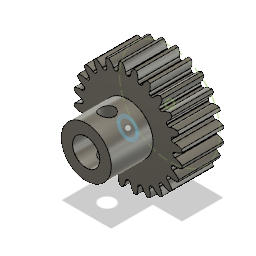
GearHægriVinstri v1 (Autodesk Fusion 360 design; units mm, degrees)
description: Spur Gear; Module: 1.000000; Num Teeth: 24; Pressure Angle: 20.000000; Backlash: 0.00 mm
Autodesk Fusion 360 part; units mm, degrees
(part 1 of 5)
sketch "Sketch1" plane through (0, 0, 0) normal (0, 0, 1) x (1, 0, 0)
  circle A0 centre (0, 0) radius 10.7492
  circle A1 centre (0, 0) radius 2
extrude "Extrude1" add sketch "Sketch1" along normal blind 2
sketch "Sketch2" plane through (0, 0, 0) normal (0, 0, 1) x (1, 0, 0)
  spline S0 degree 5 poles (11.2399, -0.9051) (11.2449, -0.9055) (11.255, -0.9062) (11.27, -0.9068) (11.2901, -0.907) (11.3152, -0.9062) (11.3404, -0.9047) (11.3655, -0.9028) (11.3907, -0.9006) (11.416, -0.8982) (11.4412, -0.8957) (11.4664, -0.8929) (11.4917, -0.8899) (11.5169, -0.8866) (11.5422, -0.8828) (11.5674, -0.8788) (11.5927, -0.8745) (11.6179, -0.87) (11.6432, -0.8652) (11.6685, -0.8603) (11.6937, -0.8552) (11.719, -0.8499) (11.7443, -0.8443) (11.7695, -0.8386) (11.7948, -0.8327) (11.82, -0.8265) (11.8453, -0.8202) (11.8706, -0.8136) (11.8958, -0.8069) (11.921, -0.8) (11.9463, -0.7929) (11.9715, -0.7857) (11.9967, -0.7783) (12.0219, -0.7707) (12.0471, -0.7629) (12.0723, -0.755) (12.0975, -0.7469) (12.1227, -0.7387) (12.1479, -0.7302) (12.173, -0.7217) (12.1982, -0.7129) (12.2233, -0.7041) (12.2484, -0.695) (12.2735, -0.6858) (12.2986, -0.6765) (12.3237, -0.667) (12.3488, -0.6573) (12.3739, -0.6475) (12.3989, -0.6376) (12.424, -0.6275) (12.449, -0.6173) (12.474, -0.6069) (12.499, -0.5964) (12.5239, -0.5858) (12.5489, -0.575) (12.5738, -0.564) (12.5988, -0.553) (12.6237, -0.5418) (12.6486, -0.5304) (12.6735, -0.5189) (12.6983, -0.5073) (12.7232, -0.4956) (12.748, -0.4837) (12.7728, -0.4717) (12.7976, -0.4595) (12.8223, -0.4473) (12.8471, -0.4349) (12.8718, -0.4223) (12.8965, -0.4097) (12.9212, -0.3969) (12.9458, -0.384) (12.9655, -0.3735) (12.9803, -0.3657) (12.9902, -0.3604) (12.9951, -0.3577) knots 0 0 0 0 0 0 0.01428571 0.02857143 0.04285714 0.05714286 0.07142857 0.08571429 0.1 0.11428571 0.12857143 0.14285714 0.15714286 0.17142857 0.18571429 0.2 0.21428571 0.22857143 0.24285714 0.25714286 0.27142857 0.28571429 0.3 0.31428571 0.32857143 0.34285714 0.35714286 0.37142857 0.38571429 0.4 0.41428571 0.42857143 0.44285714 0.45714286 0.47142857 0.48571429 0.5 0.51428571 0.52857143 0.54285714 0.55714286 0.57142857 0.58571429 0.6 0.61428571 0.62857143 0.64285714 0.65714286 0.67142857 0.68571429 0.7 0.71428571 0.72857143 0.74285714 0.75714286 0.77142857 0.78571429 0.8 0.81428571 0.82857143 0.84285714 0.85714286 0.87142857 0.88571429 0.9 0.91428571 0.92857143 0.94285714 0.95714286 0.97142857 0.98571429 1 1 1 1 1 1
  spline S1 degree 5 poles (11.2399, 0.9051) (11.2449, 0.9055) (11.255, 0.9062) (11.27, 0.9068) (11.2901, 0.907) (11.3152, 0.9062) (11.3404, 0.9047) (11.3655, 0.9028) (11.3907, 0.9006) (11.416, 0.8982) (11.4412, 0.8957) (11.4664, 0.8929) (11.4917, 0.8899) (11.5169, 0.8866) (11.5422, 0.8828) (11.5674, 0.8788) (11.5927, 0.8745) (11.6179, 0.87) (11.6432, 0.8652) (11.6685, 0.8603) (11.6937, 0.8552) (11.719, 0.8499) (11.7443, 0.8443) (11.7695, 0.8386) (11.7948, 0.8327) (11.82, 0.8265) (11.8453, 0.8202) (11.8706, 0.8136) (11.8958, 0.8069) (11.921, 0.8) (11.9463, 0.7929) (11.9715, 0.7857) (11.9967, 0.7783) (12.0219, 0.7707) (12.0471, 0.7629) (12.0723, 0.755) (12.0975, 0.7469) (12.1227, 0.7387) (12.1479, 0.7302) (12.173, 0.7217) (12.1982, 0.7129) (12.2233, 0.7041) (12.2484, 0.695) (12.2735, 0.6858) (12.2986, 0.6765) (12.3237, 0.667) (12.3488, 0.6573) (12.3739, 0.6475) (12.3989, 0.6376) (12.424, 0.6275) (12.449, 0.6173) (12.474, 0.6069) (12.499, 0.5964) (12.5239, 0.5858) (12.5489, 0.575) (12.5738, 0.564) (12.5988, 0.553) (12.6237, 0.5418) (12.6486, 0.5304) (12.6735, 0.5189) (12.6983, 0.5073) (12.7232, 0.4956) (12.748, 0.4837) (12.7728, 0.4717) (12.7976, 0.4595) (12.8223, 0.4473) (12.8471, 0.4349) (12.8718, 0.4223) (12.8965, 0.4097) (12.9212, 0.3969) (12.9458, 0.384) (12.9655, 0.3735) (12.9803, 0.3657) (12.9902, 0.3604) (12.9951, 0.3577) knots 0 0 0 0 0 0 0.01428571 0.02857143 0.04285714 0.05714286 0.07142857 0.08571429 0.1 0.11428571 0.12857143 0.14285714 0.15714286 0.17142857 0.18571429 0.2 0.21428571 0.22857143 0.24285714 0.25714286 0.27142857 0.28571429 0.3 0.31428571 0.32857143 0.34285714 0.35714286 0.37142857 0.38571429 0.4 0.41428571 0.42857143 0.44285714 0.45714286 0.47142857 0.48571429 0.5 0.51428571 0.52857143 0.54285714 0.55714286 0.57142857 0.58571429 0.6 0.61428571 0.62857143 0.64285714 0.65714286 0.67142857 0.68571429 0.7 0.71428571 0.72857143 0.74285714 0.75714286 0.77142857 0.78571429 0.8 0.81428571 0.82857143 0.84285714 0.85714286 0.87142857 0.88571429 0.9 0.91428571 0.92857143 0.94285714 0.95714286 0.97142857 0.98571429 1 1 1 1 1 1
  arc A0 (12.9951, -0.3577) -> (12.9951, 0.3577) centre (0, 0) ccw
  line L0 (10.7045, -0.8628) -> (11.2399, -0.9051)
  line L1 (10.7045, 0.8628) -> (11.2399, 0.9051)
  line L2 (10.7045, -0.8628) -> (10.7045, 0.8628)
  point P0 (11.3636, -0.9028)
  point P1 (11.4881, -0.8903)
  point P2 (11.6131, -0.8708)
  point P3 (11.7384, -0.8456)
  point P4 (11.8639, -0.8153)
  point P5 (11.9897, -0.7803)
  point P6 (12.1155, -0.741)
  point P7 (12.2414, -0.6975)
  point P8 (12.3673, -0.6501)
  point P9 (12.4932, -0.5988)
  point P10 (12.6189, -0.5439)
  point P11 (12.7445, -0.4853)
  point P12 (12.8699, -0.4232)
  point P13 (11.3636, 0.9028)
  point P14 (11.4881, 0.8903)
  point P15 (11.6131, 0.8708)
  point P16 (11.7384, 0.8456)
  point P17 (11.8639, 0.8153)
  point P18 (11.9897, 0.7803)
  point P19 (12.1155, 0.741)
  point P20 (12.2414, 0.6975)
  point P21 (12.3673, 0.6501)
  point P22 (12.4932, 0.5988)
  point P23 (12.6189, 0.5439)
  point P24 (12.7445, 0.4853)
  point P25 (12.8699, 0.4232)
extrude "Extrude2" add sketch "Sketch2" along normal blind 2
fillet "Fillet1" radius 0.5 2 edges at (10.7145, -0.8636, 1) (10.7145, 0.8636, 1)
pattern_circular "C-Pattern1" count 24 over 360 about axis through (0, 0, 0) along (0, 0, 1) of "Extrude2", "Fillet1"
sketch "Sketch3" plane through (0, 0, 0) normal (0, 0, 1) x (1, 0, 0)
  circle A0 centre (0, 0) radius 12 construction
move_body "Move1" bodies 1 to x (0.994522, -0.104528, 0) y (0.104528, 0.994522, 0) z (0, 0, 1) at (0, 0, 0)
move_body "Move2" bodies 1 to x (0.999848, -0.017452, 0) y (0.017452, 0.999848, 0) z (0, 0, 1) at (0, 0, 0)
move_body "Move3" bodies 1 to x (0.999998, -0.001745, 0) y (0.001745, 0.999998, 0) z (0, 0, 1) at (0, 0, 0)
move_body "Move4" bodies 1 to x (0.999962, -0.008727, 0) y (0.008727, 0.999962, 0) z (0, 0, 1) at (0, 0, 0)
move_body "Move5" bodies 1 to x (0.999994, 0.003491, 0) y (-0.003491, 0.999994, 0) z (0, 0, 1) at (0, 0, 0)
move_body "Move6" bodies 1 to x (0.999998, -0.001745, 0) y (0.001745, 0.999998, 0) z (0, 0, 1) at (0, 0, 0)
extrude "Extrude3" add 1 faces at (4.7398, 6.177, 2) along direction (0, 0, 1) blind 8
sketch "sketch 2008" plane through (-156.112, -54.0793, 10) normal (0, 0, 1) x (-1, 0, 0)
  circle A0 centre (-156.112, -54.0793) radius 2
  circle A1 centre (-156.112, -54.0793) radius 2.45
extrude "Extrude4" cut sketch "sketch 2008" against normal blind 50
sketch "sketch 2024" plane through (-92.8019, -19.9804, 10) normal (0, 0, 1) x (-1, 0, 0)
  circle A0 centre (-92.8019, -19.9804) radius 2.45
  circle A1 centre (-92.8019, -19.9804) radius 2.475
extrude "Extrude5" cut sketch "sketch 2024" against normal blind 20
sketch "Sketch4" plane through (0, 0, 10) normal (0, 0, 1) x (1, 0, 0)
  circle A0 centre (0, 0) radius 2.475
  arc A1 (10.3658, -2.8452) -> (10.3996, -2.7189) centre (0, 0) ccw
  arc A2 (10.9875, -2.3564) -> (10.3996, -2.7189) centre (10.8834, -2.8454) ccw
  line L0 (10.9875, -2.3564) -> (11.0256, -2.3645)
  spline S0 degree 5 poles (11.0256, -2.3645) (11.0305, -2.3655) (11.0404, -2.3675) (11.0552, -2.3701) (11.0751, -2.3729) (11.1001, -2.3754) (11.1253, -2.3772) (11.1505, -2.3785) (11.1757, -2.3797) (11.201, -2.3806) (11.2264, -2.3814) (11.2518, -2.382) (11.2772, -2.3823) (11.3027, -2.3822) (11.3282, -2.3818) (11.3537, -2.3811) (11.3793, -2.3802) (11.405, -2.379) (11.4307, -2.3776) (11.4564, -2.376) (11.4821, -2.3742) (11.5078, -2.3722) (11.5336, -2.3701) (11.5594, -2.3677) (11.5852, -2.3651) (11.611, -2.3623) (11.6369, -2.3593) (11.6628, -2.3561) (11.6887, -2.3527) (11.7146, -2.3492) (11.7406, -2.3455) (11.7665, -2.3416) (11.7925, -2.3375) (11.8185, -2.3333) (11.8445, -2.3289) (11.8705, -2.3243) (11.8965, -2.3196) (11.9226, -2.3147) (11.9486, -2.3096) (11.9747, -2.3044) (12.0007, -2.299) (12.0268, -2.2935) (12.0529, -2.2878) (12.079, -2.282) (12.1051, -2.276) (12.1312, -2.2698) (12.1574, -2.2636) (12.1835, -2.2571) (12.2096, -2.2505) (12.2358, -2.2438) (12.2619, -2.2369) (12.288, -2.2299) (12.3142, -2.2227) (12.3403, -2.2154) (12.3665, -2.208) (12.3927, -2.2004) (12.4188, -2.1927) (12.445, -2.1848) (12.4711, -2.1768) (12.4973, -2.1687) (12.5235, -2.1604) (12.5496, -2.152) (12.5758, -2.1435) (12.6019, -2.1348) (12.6281, -2.126) (12.6542, -2.1171) (12.6804, -2.108) (12.7065, -2.0988) (12.7327, -2.0895) (12.7588, -2.08) (12.785, -2.0705) (12.8059, -2.0627) (12.8215, -2.0568) (12.832, -2.0528) (12.8372, -2.0509) knots 0 0 0 0 0 0 0.01428571 0.02857143 0.04285714 0.05714286 0.07142857 0.08571429 0.1 0.11428571 0.12857143 0.14285714 0.15714286 0.17142857 0.18571429 0.2 0.21428571 0.22857143 0.24285714 0.25714286 0.27142857 0.28571429 0.3 0.31428571 0.32857143 0.34285714 0.35714286 0.37142857 0.38571429 0.4 0.41428571 0.42857143 0.44285714 0.45714286 0.47142857 0.48571429 0.5 0.51428571 0.52857143 0.54285714 0.55714286 0.57142857 0.58571429 0.6 0.61428571 0.62857143 0.64285714 0.65714286 0.67142857 0.68571429 0.7 0.71428571 0.72857143 0.74285714 0.75714286 0.77142857 0.78571429 0.8 0.81428571 0.82857143 0.84285714 0.85714286 0.87142857 0.88571429 0.9 0.91428571 0.92857143 0.94285714 0.95714286 0.97142857 0.98571429 1 1 1 1 1 1
  arc A3 (12.8372, -2.0509) -> (12.9306, -1.3415) centre (0, 0) ccw
  spline S1 degree 5 poles (12.9306, -1.3415) (12.9261, -1.3383) (12.917, -1.3317) (12.9034, -1.322) (12.8852, -1.3091) (12.8624, -1.2931) (12.8396, -1.2772) (12.8168, -1.2614) (12.7939, -1.2457) (12.771, -1.2302) (12.7481, -1.2148) (12.7251, -1.1995) (12.702, -1.1844) (12.679, -1.1694) (12.6559, -1.1545) (12.6328, -1.1397) (12.6096, -1.1251) (12.5864, -1.1106) (12.5632, -1.0962) (12.5399, -1.082) (12.5166, -1.0679) (12.4933, -1.054) (12.4699, -1.0401) (12.4465, -1.0265) (12.423, -1.0129) (12.3996, -0.9995) (12.3761, -0.9862) (12.3525, -0.9731) (12.329, -0.9601) (12.3054, -0.9473) (12.2817, -0.9346) (12.2581, -0.9221) (12.2344, -0.9097) (12.2106, -0.8974) (12.1869, -0.8853) (12.1631, -0.8734) (12.1392, -0.8616) (12.1154, -0.85) (12.0915, -0.8385) (12.0676, -0.8272) (12.0436, -0.8161) (12.0197, -0.8051) (11.9957, -0.7943) (11.9716, -0.7836) (11.9476, -0.7731) (11.9235, -0.7628) (11.8993, -0.7527) (11.8752, -0.7428) (11.851, -0.733) (11.8268, -0.7234) (11.8026, -0.714) (11.7783, -0.7048) (11.754, -0.6958) (11.7297, -0.687) (11.7053, -0.6785) (11.6809, -0.6701) (11.6565, -0.6619) (11.6321, -0.6539) (11.6076, -0.6461) (11.5832, -0.6386) (11.5586, -0.6313) (11.5341, -0.6243) (11.5095, -0.6177) (11.4849, -0.6114) (11.4602, -0.6053) (11.4355, -0.5996) (11.4108, -0.5939) (11.3861, -0.5885) (11.3614, -0.5833) (11.3367, -0.5785) (11.3119, -0.5744) (11.2919, -0.572) (11.2769, -0.5706) (11.2669, -0.57) (11.2619, -0.5697) knots -1 -1 -1 -1 -1 -1 -0.98571429 -0.97142857 -0.95714286 -0.94285714 -0.92857143 -0.91428571 -0.9 -0.88571429 -0.87142857 -0.85714286 -0.84285714 -0.82857143 -0.81428571 -0.8 -0.78571429 -0.77142857 -0.75714286 -0.74285714 -0.72857143 -0.71428571 -0.7 -0.68571429 -0.67142857 -0.65714286 -0.64285714 -0.62857143 -0.61428571 -0.6 -0.58571429 -0.57142857 -0.55714286 -0.54285714 -0.52857143 -0.51428571 -0.5 -0.48571429 -0.47142857 -0.45714286 -0.44285714 -0.42857143 -0.41428571 -0.4 -0.38571429 -0.37142857 -0.35714286 -0.34285714 -0.32857143 -0.31428571 -0.3 -0.28571429 -0.27142857 -0.25714286 -0.24285714 -0.22857143 -0.21428571 -0.2 -0.18571429 -0.17142857 -0.15714286 -0.14285714 -0.12857143 -0.11428571 -0.1 -0.08571429 -0.07142857 -0.05714286 -0.04285714 -0.02857143 -0.01428571 0 0 0 0 0 0
  line L1 (11.2619, -0.5697) -> (11.223, -0.5677)
  arc A4 (10.749, -0.0653) -> (11.223, -0.5677) centre (11.249, -0.0684) ccw
  arc A5 (10.749, -0.0653) -> (10.749, 0.0653) centre (0, 0) ccw
  arc A6 (11.223, 0.5677) -> (10.749, 0.0653) centre (11.249, 0.0684) ccw
  line L2 (11.223, 0.5677) -> (11.2619, 0.5697)
  spline S2 degree 5 poles (11.2619, 0.5697) (11.2669, 0.57) (11.2769, 0.5706) (11.2919, 0.572) (11.3119, 0.5744) (11.3367, 0.5785) (11.3614, 0.5833) (11.3861, 0.5885) (11.4108, 0.5939) (11.4355, 0.5996) (11.4602, 0.6053) (11.4849, 0.6114) (11.5095, 0.6177) (11.5341, 0.6243) (11.5586, 0.6313) (11.5832, 0.6386) (11.6076, 0.6461) (11.6321, 0.6539) (11.6565, 0.6619) (11.6809, 0.6701) (11.7053, 0.6785) (11.7297, 0.687) (11.754, 0.6958) (11.7783, 0.7048) (11.8026, 0.714) (11.8268, 0.7234) (11.851, 0.733) (11.8752, 0.7428) (11.8993, 0.7527) (11.9235, 0.7628) (11.9476, 0.7731) (11.9716, 0.7836) (11.9957, 0.7943) (12.0197, 0.8051) (12.0436, 0.8161) (12.0676, 0.8272) (12.0915, 0.8385) (12.1154, 0.85) (12.1392, 0.8616) (12.1631, 0.8734) (12.1869, 0.8853) (12.2106, 0.8974) (12.2344, 0.9097) (12.2581, 0.9221) (12.2817, 0.9346) (12.3054, 0.9473) (12.329, 0.9601) (12.3525, 0.9731) (12.3761, 0.9862) (12.3996, 0.9995) (12.423, 1.0129) (12.4465, 1.0265) (12.4699, 1.0401) (12.4933, 1.054) (12.5166, 1.0679) (12.5399, 1.082) (12.5632, 1.0962) (12.5864, 1.1106) (12.6096, 1.1251) (12.6328, 1.1397) (12.6559, 1.1545) (12.679, 1.1694) (12.702, 1.1844) (12.7251, 1.1995) (12.7481, 1.2148) (12.771, 1.2302) (12.7939, 1.2457) (12.8168, 1.2614) (12.8396, 1.2772) (12.8624, 1.2931) (12.8852, 1.3091) (12.9034, 1.322) (12.917, 1.3317) (12.9261, 1.3383) (12.9306, 1.3415) knots 0 0 0 0 0 0 0.01428571 0.02857143 0.04285714 0.05714286 0.07142857 0.08571429 0.1 0.11428571 0.12857143 0.14285714 0.15714286 0.17142857 0.18571429 0.2 0.21428571 0.22857143 0.24285714 0.25714286 0.27142857 0.28571429 0.3 0.31428571 0.32857143 0.34285714 0.35714286 0.37142857 0.38571429 0.4 0.41428571 0.42857143 0.44285714 0.45714286 0.47142857 0.48571429 0.5 0.51428571 0.52857143 0.54285714 0.55714286 0.57142857 0.58571429 0.6 0.61428571 0.62857143 0.64285714 0.65714286 0.67142857 0.68571429 0.7 0.71428571 0.72857143 0.74285714 0.75714286 0.77142857 0.78571429 0.8 0.81428571 0.82857143 0.84285714 0.85714286 0.87142857 0.88571429 0.9 0.91428571 0.92857143 0.94285714 0.95714286 0.97142857 0.98571429 1 1 1 1 1 1
  arc A7 (12.9306, 1.3415) -> (12.8372, 2.0509) centre (0, 0) ccw
  spline S3 degree 5 poles (12.8372, 2.0509) (12.832, 2.0528) (12.8215, 2.0568) (12.8059, 2.0627) (12.785, 2.0705) (12.7588, 2.08) (12.7327, 2.0895) (12.7065, 2.0988) (12.6804, 2.108) (12.6542, 2.1171) (12.6281, 2.126) (12.6019, 2.1348) (12.5758, 2.1435) (12.5496, 2.152) (12.5235, 2.1604) (12.4973, 2.1687) (12.4711, 2.1768) (12.445, 2.1848) (12.4188, 2.1927) (12.3927, 2.2004) (12.3665, 2.208) (12.3403, 2.2154) (12.3142, 2.2227) (12.288, 2.2299) (12.2619, 2.2369) (12.2358, 2.2438) (12.2096, 2.2505) (12.1835, 2.2571) (12.1574, 2.2636) (12.1312, 2.2698) (12.1051, 2.276) (12.079, 2.282) (12.0529, 2.2878) (12.0268, 2.2935) (12.0007, 2.299) (11.9747, 2.3044) (11.9486, 2.3096) (11.9226, 2.3147) (11.8965, 2.3196) (11.8705, 2.3243) (11.8445, 2.3289) (11.8185, 2.3333) (11.7925, 2.3375) (11.7665, 2.3416) (11.7406, 2.3455) (11.7146, 2.3492) (11.6887, 2.3527) (11.6628, 2.3561) (11.6369, 2.3593) (11.611, 2.3623) (11.5852, 2.3651) (11.5594, 2.3677) (11.5336, 2.3701) (11.5078, 2.3722) (11.4821, 2.3742) (11.4564, 2.376) (11.4307, 2.3776) (11.405, 2.379) (11.3793, 2.3802) (11.3537, 2.3811) (11.3282, 2.3818) (11.3027, 2.3822) (11.2772, 2.3823) (11.2518, 2.382) (11.2264, 2.3814) (11.201, 2.3806) (11.1757, 2.3797) (11.1505, 2.3785) (11.1253, 2.3772) (11.1001, 2.3754) (11.0751, 2.3729) (11.0552, 2.3701) (11.0404, 2.3675) (11.0305, 2.3655) (11.0256, 2.3645) knots -1 -1 -1 -1 -1 -1 -0.98571429 -0.97142857 -0.95714286 -0.94285714 -0.92857143 -0.91428571 -0.9 -0.88571429 -0.87142857 -0.85714286 -0.84285714 -0.82857143 -0.81428571 -0.8 -0.78571429 -0.77142857 -0.75714286 -0.74285714 -0.72857143 -0.71428571 -0.7 -0.68571429 -0.67142857 -0.65714286 -0.64285714 -0.62857143 -0.61428571 -0.6 -0.58571429 -0.57142857 -0.55714286 -0.54285714 -0.52857143 -0.51428571 -0.5 -0.48571429 -0.47142857 -0.45714286 -0.44285714 -0.42857143 -0.41428571 -0.4 -0.38571429 -0.37142857 -0.35714286 -0.34285714 -0.32857143 -0.31428571 -0.3 -0.28571429 -0.27142857 -0.25714286 -0.24285714 -0.22857143 -0.21428571 -0.2 -0.18571429 -0.17142857 -0.15714286 -0.14285714 -0.12857143 -0.11428571 -0.1 -0.08571429 -0.07142857 -0.05714286 -0.04285714 -0.02857143 -0.01428571 0 0 0 0 0 0
  line L3 (11.0256, 2.3645) -> (10.9875, 2.3564)
  arc A8 (10.3996, 2.7189) -> (10.9875, 2.3564) centre (10.8834, 2.8454) ccw
  arc A9 (10.3996, 2.7189) -> (10.3658, 2.8452) centre (0, 0) ccw
  arc A10 (10.6936, 3.4531) -> (10.3658, 2.8452) centre (10.848, 2.9775) ccw
  line L4 (10.6936, 3.4531) -> (10.7307, 3.4651)
  spline S4 degree 5 poles (10.7307, 3.4651) (10.7355, 3.4667) (10.745, 3.4699) (10.7591, 3.475) (10.7777, 3.4826) (10.8007, 3.4929) (10.8233, 3.5039) (10.8459, 3.5154) (10.8683, 3.527) (10.8907, 3.5389) (10.913, 3.5508) (10.9353, 3.563) (10.9575, 3.5755) (10.9795, 3.5883) (11.0014, 3.6013) (11.0232, 3.6147) (11.0449, 3.6284) (11.0665, 3.6422) (11.088, 3.6563) (11.1095, 3.6705) (11.1309, 3.6849) (11.1522, 3.6995) (11.1734, 3.7143) (11.1946, 3.7292) (11.2156, 3.7444) (11.2366, 3.7597) (11.2575, 3.7753) (11.2783, 3.791) (11.2991, 3.8068) (11.3197, 3.8229) (11.3404, 3.8391) (11.3609, 3.8554) (11.3814, 3.8719) (11.4017, 3.8886) (11.4221, 3.9054) (11.4423, 3.9223) (11.4625, 3.9395) (11.4826, 3.9567) (11.5026, 3.9741) (11.5226, 3.9917) (11.5425, 4.0094) (11.5623, 4.0272) (11.582, 4.0452) (11.6017, 4.0633) (11.6213, 4.0815) (11.6409, 4.0999) (11.6604, 4.1184) (11.6798, 4.137) (11.6991, 4.1558) (11.7184, 4.1747) (11.7376, 4.1937) (11.7567, 4.2129) (11.7758, 4.2321) (11.7948, 4.2515) (11.8137, 4.2711) (11.8326, 4.2907) (11.8514, 4.3105) (11.8701, 4.3304) (11.8887, 4.3504) (11.9073, 4.3705) (11.9259, 4.3907) (11.9443, 4.4111) (11.9627, 4.4316) (11.981, 4.4522) (11.9993, 4.4729) (12.0174, 4.4937) (12.0356, 4.5146) (12.0536, 4.5356) (12.0716, 4.5568) (12.0895, 4.578) (12.1073, 4.5994) (12.1215, 4.6166) (12.1322, 4.6295) (12.1392, 4.6382) (12.1428, 4.6425) knots 0 0 0 0 0 0 0.01428571 0.02857143 0.04285714 0.05714286 0.07142857 0.08571429 0.1 0.11428571 0.12857143 0.14285714 0.15714286 0.17142857 0.18571429 0.2 0.21428571 0.22857143 0.24285714 0.25714286 0.27142857 0.28571429 0.3 0.31428571 0.32857143 0.34285714 0.35714286 0.37142857 0.38571429 0.4 0.41428571 0.42857143 0.44285714 0.45714286 0.47142857 0.48571429 0.5 0.51428571 0.52857143 0.54285714 0.55714286 0.57142857 0.58571429 0.6 0.61428571 0.62857143 0.64285714 0.65714286 0.67142857 0.68571429 0.7 0.71428571 0.72857143 0.74285714 0.75714286 0.77142857 0.78571429 0.8 0.81428571 0.82857143 0.84285714 0.85714286 0.87142857 0.88571429 0.9 0.91428571 0.92857143 0.94285714 0.95714286 0.97142857 0.98571429 1 1 1 1 1 1
  arc A11 (12.1428, 4.6425) -> (11.869, 5.3035) centre (0, 0) ccw
  spline S5 degree 5 poles (11.869, 5.3035) (11.8634, 5.3041) (11.8523, 5.3052) (11.8356, 5.3068) (11.8134, 5.3089) (11.7857, 5.3114) (11.758, 5.3138) (11.7304, 5.316) (11.7027, 5.3181) (11.6751, 5.3201) (11.6475, 5.322) (11.62, 5.3237) (11.5925, 5.3253) (11.565, 5.3268) (11.5376, 5.3281) (11.5102, 5.3293) (11.4828, 5.3304) (11.4554, 5.3314) (11.4281, 5.3322) (11.4009, 5.3329) (11.3736, 5.3335) (11.3465, 5.3339) (11.3193, 5.3342) (11.2922, 5.3343) (11.2651, 5.3343) (11.2381, 5.3342) (11.2111, 5.3339) (11.1842, 5.3335) (11.1573, 5.333) (11.1304, 5.3323) (11.1036, 5.3315) (11.0768, 5.3305) (11.0501, 5.3294) (11.0234, 5.3281) (10.9968, 5.3267) (10.9702, 5.3252) (10.9437, 5.3234) (10.9172, 5.3216) (10.8908, 5.3196) (10.8644, 5.3174) (10.8381, 5.3151) (10.8119, 5.3126) (10.7857, 5.31) (10.7595, 5.3072) (10.7335, 5.3042) (10.7075, 5.3011) (10.6815, 5.2978) (10.6556, 5.2943) (10.6298, 5.2907) (10.604, 5.2869) (10.5783, 5.283) (10.5527, 5.2788) (10.5272, 5.2744) (10.5017, 5.2698) (10.4763, 5.2651) (10.451, 5.2601) (10.4258, 5.255) (10.4007, 5.2497) (10.3756, 5.2443) (10.3506, 5.2386) (10.3257, 5.2326) (10.301, 5.2264) (10.2763, 5.2198) (10.2519, 5.213) (10.2275, 5.2059) (10.2032, 5.1985) (10.179, 5.1911) (10.1549, 5.1834) (10.1309, 5.1756) (10.1071, 5.1673) (10.0836, 5.1585) (10.0651, 5.1506) (10.0514, 5.1443) (10.0424, 5.1398) (10.038, 5.1376) knots -1 -1 -1 -1 -1 -1 -0.98571429 -0.97142857 -0.95714286 -0.94285714 -0.92857143 -0.91428571 -0.9 -0.88571429 -0.87142857 -0.85714286 -0.84285714 -0.82857143 -0.81428571 -0.8 -0.78571429 -0.77142857 -0.75714286 -0.74285714 -0.72857143 -0.71428571 -0.7 -0.68571429 -0.67142857 -0.65714286 -0.64285714 -0.62857143 -0.61428571 -0.6 -0.58571429 -0.57142857 -0.55714286 -0.54285714 -0.52857143 -0.51428571 -0.5 -0.48571429 -0.47142857 -0.45714286 -0.44285714 -0.42857143 -0.41428571 -0.4 -0.38571429 -0.37142857 -0.35714286 -0.34285714 -0.32857143 -0.31428571 -0.3 -0.28571429 -0.27142857 -0.25714286 -0.24285714 -0.22857143 -0.21428571 -0.2 -0.18571429 -0.17142857 -0.15714286 -0.14285714 -0.12857143 -0.11428571 -0.1 -0.08571429 -0.07142857 -0.05714286 -0.04285714 -0.02857143 -0.01428571 0 0 0 0 0 0
  line L5 (10.038, 5.1376) -> (10.0032, 5.1199)
  arc A12 (9.3416, 5.3179) -> (10.0032, 5.1199) centre (9.7761, 5.5653) ccw
  arc A13 (9.3416, 5.3179) -> (9.2762, 5.4311) centre (0, 0) ccw
  arc A14 (9.4355, 6.1031) -> (9.2762, 5.4311) centre (9.7077, 5.6837) ccw
  line L6 (9.4355, 6.1031) -> (9.4682, 6.1244)
  spline S6 degree 5 poles (9.4682, 6.1244) (9.4725, 6.1271) (9.4808, 6.1327) (9.4931, 6.1413) (9.5091, 6.1534) (9.5286, 6.1693) (9.5477, 6.1858) (9.5665, 6.2027) (9.5851, 6.2198) (9.6037, 6.237) (9.6222, 6.2543) (9.6405, 6.2719) (9.6587, 6.2897) (9.6767, 6.3077) (9.6944, 6.326) (9.712, 6.3446) (9.7295, 6.3634) (9.7467, 6.3824) (9.7639, 6.4015) (9.7809, 6.4208) (9.7979, 6.4402) (9.8147, 6.4598) (9.8314, 6.4796) (9.8479, 6.4995) (9.8643, 6.5196) (9.8806, 6.5399) (9.8968, 6.5603) (9.9128, 6.5809) (9.9288, 6.6015) (9.9446, 6.6224) (9.9603, 6.6433) (9.9759, 6.6644) (9.9914, 6.6857) (10.0068, 6.707) (10.0221, 6.7285) (10.0372, 6.7502) (10.0523, 6.7719) (10.0672, 6.7938) (10.0821, 6.8158) (10.0968, 6.8379) (10.1115, 6.8602) (10.126, 6.8825) (10.1404, 6.905) (10.1548, 6.9276) (10.169, 6.9503) (10.1831, 6.9731) (10.1971, 6.996) (10.211, 7.019) (10.2249, 7.0421) (10.2386, 7.0654) (10.2522, 7.0887) (10.2657, 7.1122) (10.2792, 7.1357) (10.2925, 7.1594) (10.3057, 7.1831) (10.3189, 7.207) (10.3319, 7.231) (10.3448, 7.255) (10.3577, 7.2792) (10.3704, 7.3034) (10.3831, 7.3278) (10.3956, 7.3522) (10.4081, 7.3767) (10.4205, 7.4014) (10.4327, 7.4261) (10.4449, 7.4509) (10.457, 7.4758) (10.469, 7.5008) (10.4809, 7.5259) (10.4927, 7.551) (10.5044, 7.5763) (10.5136, 7.5966) (10.5206, 7.6118) (10.5252, 7.622) (10.5275, 7.6271) knots 0 0 0 0 0 0 0.01428571 0.02857143 0.04285714 0.05714286 0.07142857 0.08571429 0.1 0.11428571 0.12857143 0.14285714 0.15714286 0.17142857 0.18571429 0.2 0.21428571 0.22857143 0.24285714 0.25714286 0.27142857 0.28571429 0.3 0.31428571 0.32857143 0.34285714 0.35714286 0.37142857 0.38571429 0.4 0.41428571 0.42857143 0.44285714 0.45714286 0.47142857 0.48571429 0.5 0.51428571 0.52857143 0.54285714 0.55714286 0.57142857 0.58571429 0.6 0.61428571 0.62857143 0.64285714 0.65714286 0.67142857 0.68571429 0.7 0.71428571 0.72857143 0.74285714 0.75714286 0.77142857 0.78571429 0.8 0.81428571 0.82857143 0.84285714 0.85714286 0.87142857 0.88571429 0.9 0.91428571 0.92857143 0.94285714 0.95714286 0.97142857 0.98571429 1 1 1 1 1 1
  arc A15 (10.5275, 7.6271) -> (10.0919, 8.1947) centre (0, 0) ccw
  spline S7 degree 5 poles (10.0919, 8.1947) (10.0864, 8.1938) (10.0754, 8.192) (10.0589, 8.1893) (10.0369, 8.1855) (10.0094, 8.1808) (9.9821, 8.1759) (9.9548, 8.1709) (9.9275, 8.1658) (9.9004, 8.1606) (9.8732, 8.1552) (9.8462, 8.1498) (9.8192, 8.1442) (9.7923, 8.1385) (9.7654, 8.1327) (9.7386, 8.1268) (9.7119, 8.1208) (9.6852, 8.1146) (9.6587, 8.1083) (9.6321, 8.1019) (9.6057, 8.0954) (9.5793, 8.0888) (9.553, 8.0821) (9.5268, 8.0752) (9.5007, 8.0682) (9.4746, 8.0611) (9.4486, 8.0538) (9.4227, 8.0465) (9.3968, 8.039) (9.371, 8.0314) (9.3454, 8.0236) (9.3197, 8.0158) (9.2942, 8.0078) (9.2688, 7.9996) (9.2434, 7.9914) (9.2182, 7.983) (9.193, 7.9745) (9.1679, 7.9658) (9.1429, 7.9571) (9.118, 7.9482) (9.0932, 7.9391) (9.0685, 7.9299) (9.0438, 7.9206) (9.0193, 7.9111) (8.9949, 7.9015) (8.9706, 7.8918) (8.9464, 7.8819) (8.9222, 7.8718) (8.8982, 7.8616) (8.8743, 7.8513) (8.8505, 7.8408) (8.8269, 7.8302) (8.8033, 7.8193) (8.7799, 7.8083) (8.7567, 7.7972) (8.7335, 7.7858) (8.7105, 7.7744) (8.6875, 7.7627) (8.6647, 7.751) (8.6421, 7.739) (8.6196, 7.7268) (8.5973, 7.7144) (8.5752, 7.7017) (8.5533, 7.6887) (8.5316, 7.6755) (8.5101, 7.6622) (8.4887, 7.6487) (8.4673, 7.6351) (8.4462, 7.6213) (8.4253, 7.6072) (8.4049, 7.5925) (8.389, 7.5802) (8.3775, 7.5705) (8.37, 7.5639) (8.3662, 7.5605) knots -1 -1 -1 -1 -1 -1 -0.98571429 -0.97142857 -0.95714286 -0.94285714 -0.92857143 -0.91428571 -0.9 -0.88571429 -0.87142857 -0.85714286 -0.84285714 -0.82857143 -0.81428571 -0.8 -0.78571429 -0.77142857 -0.75714286 -0.74285714 -0.72857143 -0.71428571 -0.7 -0.68571429 -0.67142857 -0.65714286 -0.64285714 -0.62857143 -0.61428571 -0.6 -0.58571429 -0.57142857 -0.55714286 -0.54285714 -0.52857143 -0.51428571 -0.5 -0.48571429 -0.47142857 -0.45714286 -0.44285714 -0.42857143 -0.41428571 -0.4 -0.38571429 -0.37142857 -0.35714286 -0.34285714 -0.32857143 -0.31428571 -0.3 -0.28571429 -0.27142857 -0.25714286 -0.24285714 -0.22857143 -0.21428571 -0.2 -0.18571429 -0.17142857 -0.15714286 -0.14285714 -0.12857143 -0.11428571 -0.1 -0.08571429 -0.07142857 -0.05714286 -0.04285714 -0.02857143 -0.01428571 0 0 0 0 0 0
  line L7 (8.3662, 7.5605) -> (8.3373, 7.5344)
  arc A16 (7.6469, 7.5545) -> (8.3373, 7.5344) centre (8.0026, 7.9059) ccw
  arc A17 (7.6469, 7.5545) -> (7.5545, 7.6469) centre (0, 0) ccw
  arc A18 (7.5344, 8.3373) -> (7.5545, 7.6469) centre (7.9059, 8.0026) ccw
  line L8 (7.5344, 8.3373) -> (7.5605, 8.3662)
  spline S8 degree 5 poles (7.5605, 8.3662) (7.5639, 8.37) (7.5705, 8.3775) (7.5802, 8.389) (7.5925, 8.4049) (7.6072, 8.4253) (7.6213, 8.4462) (7.6351, 8.4673) (7.6487, 8.4887) (7.6622, 8.5101) (7.6755, 8.5316) (7.6887, 8.5533) (7.7017, 8.5752) (7.7144, 8.5973) (7.7268, 8.6196) (7.739, 8.6421) (7.751, 8.6647) (7.7627, 8.6875) (7.7744, 8.7105) (7.7858, 8.7335) (7.7972, 8.7567) (7.8083, 8.7799) (7.8193, 8.8033) (7.8302, 8.8269) (7.8408, 8.8505) (7.8513, 8.8743) (7.8616, 8.8982) (7.8718, 8.9222) (7.8819, 8.9464) (7.8918, 8.9706) (7.9015, 8.9949) (7.9111, 9.0193) (7.9206, 9.0438) (7.9299, 9.0685) (7.9391, 9.0932) (7.9482, 9.118) (7.9571, 9.1429) (7.9658, 9.1679) (7.9745, 9.193) (7.983, 9.2182) (7.9914, 9.2434) (7.9996, 9.2688) (8.0078, 9.2942) (8.0158, 9.3197) (8.0236, 9.3454) (8.0314, 9.371) (8.039, 9.3968) (8.0465, 9.4227) (8.0538, 9.4486) (8.0611, 9.4746) (8.0682, 9.5007) (8.0752, 9.5268) (8.0821, 9.553) (8.0888, 9.5793) (8.0954, 9.6057) (8.1019, 9.6321) (8.1083, 9.6587) (8.1146, 9.6852) (8.1208, 9.7119) (8.1268, 9.7386) (8.1327, 9.7654) (8.1385, 9.7923) (8.1442, 9.8192) (8.1498, 9.8462) (8.1552, 9.8732) (8.1606, 9.9004) (8.1658, 9.9275) (8.1709, 9.9548) (8.1759, 9.9821) (8.1808, 10.0094) (8.1855, 10.0369) (8.1893, 10.0589) (8.192, 10.0754) (8.1938, 10.0864) (8.1947, 10.0919) knots 0 0 0 0 0 0 0.01428571 0.02857143 0.04285714 0.05714286 0.07142857 0.08571429 0.1 0.11428571 0.12857143 0.14285714 0.15714286 0.17142857 0.18571429 0.2 0.21428571 0.22857143 0.24285714 0.25714286 0.27142857 0.28571429 0.3 0.31428571 0.32857143 0.34285714 0.35714286 0.37142857 0.38571429 0.4 0.41428571 0.42857143 0.44285714 0.45714286 0.47142857 0.48571429 0.5 0.51428571 0.52857143 0.54285714 0.55714286 0.57142857 0.58571429 0.6 0.61428571 0.62857143 0.64285714 0.65714286 0.67142857 0.68571429 0.7 0.71428571 0.72857143 0.74285714 0.75714286 0.77142857 0.78571429 0.8 0.81428571 0.82857143 0.84285714 0.85714286 0.87142857 0.88571429 0.9 0.91428571 0.92857143 0.94285714 0.95714286 0.97142857 0.98571429 1 1 1 1 1 1
  arc A19 (8.1947, 10.0919) -> (7.6271, 10.5275) centre (0, 0) ccw
  spline S9 degree 5 poles (7.6271, 10.5275) (7.622, 10.5252) (7.6118, 10.5206) (7.5966, 10.5136) (7.5763, 10.5044) (7.551, 10.4927) (7.5259, 10.4809) (7.5008, 10.469) (7.4758, 10.457) (7.4509, 10.4449) (7.4261, 10.4327) (7.4014, 10.4205) (7.3767, 10.4081) (7.3522, 10.3956) (7.3278, 10.3831) (7.3034, 10.3704) (7.2792, 10.3577) (7.255, 10.3448) (7.231, 10.3319) (7.207, 10.3189) (7.1831, 10.3057) (7.1594, 10.2925) (7.1357, 10.2792) (7.1122, 10.2657) (7.0887, 10.2522) (7.0654, 10.2386) (7.0421, 10.2249) (7.019, 10.211) (6.996, 10.1971) (6.9731, 10.1831) (6.9503, 10.169) (6.9276, 10.1548) (6.905, 10.1404) (6.8825, 10.126) (6.8602, 10.1115) (6.8379, 10.0968) (6.8158, 10.0821) (6.7938, 10.0672) (6.7719, 10.0523) (6.7502, 10.0372) (6.7285, 10.0221) (6.707, 10.0068) (6.6857, 9.9914) (6.6644, 9.9759) (6.6433, 9.9603) (6.6224, 9.9446) (6.6015, 9.9288) (6.5809, 9.9128) (6.5603, 9.8968) (6.5399, 9.8806) (6.5196, 9.8643) (6.4995, 9.8479) (6.4796, 9.8314) (6.4598, 9.8147) (6.4402, 9.7979) (6.4208, 9.7809) (6.4015, 9.7639) (6.3824, 9.7467) (6.3634, 9.7295) (6.3446, 9.712) (6.326, 9.6944) (6.3077, 9.6767) (6.2897, 9.6587) (6.2719, 9.6405) (6.2543, 9.6222) (6.237, 9.6037) (6.2198, 9.5851) (6.2027, 9.5665) (6.1858, 9.5477) (6.1693, 9.5286) (6.1534, 9.5091) (6.1413, 9.4931) (6.1327, 9.4808) (6.1271, 9.4725) (6.1244, 9.4682) knots -1 -1 -1 -1 -1 -1 -0.98571429 -0.97142857 -0.95714286 -0.94285714 -0.92857143 -0.91428571 -0.9 -0.88571429 -0.87142857 -0.85714286 -0.84285714 -0.82857143 -0.81428571 -0.8 -0.78571429 -0.77142857 -0.75714286 -0.74285714 -0.72857143 -0.71428571 -0.7 -0.68571429 -0.67142857 -0.65714286 -0.64285714 -0.62857143 -0.61428571 -0.6 -0.58571429 -0.57142857 -0.55714286 -0.54285714 -0.52857143 -0.51428571 -0.5 -0.48571429 -0.47142857 -0.45714286 -0.44285714 -0.42857143 -0.41428571 -0.4 -0.38571429 -0.37142857 -0.35714286 -0.34285714 -0.32857143 -0.31428571 -0.3 -0.28571429 -0.27142857 -0.25714286 -0.24285714 -0.22857143 -0.21428571 -0.2 -0.18571429 -0.17142857 -0.15714286 -0.14285714 -0.12857143 -0.11428571 -0.1 -0.08571429 -0.07142857 -0.05714286 -0.04285714 -0.02857143 -0.01428571 0 0 0 0 0 0
  line L9 (6.1244, 9.4682) -> (6.1031, 9.4355)
  arc A20 (5.4311, 9.2762) -> (6.1031, 9.4355) centre (5.6837, 9.7077) ccw
  arc A21 (5.4311, 9.2762) -> (5.3179, 9.3416) centre (0, 0) ccw
  arc A22 (5.1199, 10.0032) -> (5.3179, 9.3416) centre (5.5653, 9.7761) ccw
  line L10 (5.1199, 10.0032) -> (5.1376, 10.038)
  spline S10 degree 5 poles (5.1376, 10.038) (5.1398, 10.0424) (5.1443, 10.0514) (5.1506, 10.0651) (5.1585, 10.0836) (5.1673, 10.1071) (5.1756, 10.1309) (5.1834, 10.1549) (5.1911, 10.179) (5.1985, 10.2032) (5.2059, 10.2275) (5.213, 10.2519) (5.2198, 10.2763) (5.2264, 10.301) (5.2326, 10.3257) (5.2386, 10.3506) (5.2443, 10.3756) (5.2497, 10.4007) (5.255, 10.4258) (5.2601, 10.451) (5.2651, 10.4763) (5.2698, 10.5017) (5.2744, 10.5272) (5.2788, 10.5527) (5.283, 10.5783) (5.2869, 10.604) (5.2907, 10.6298) (5.2943, 10.6556) (5.2978, 10.6815) (5.3011, 10.7075) (5.3042, 10.7335) (5.3072, 10.7595) (5.31, 10.7857) (5.3126, 10.8119) (5.3151, 10.8381) (5.3174, 10.8644) (5.3196, 10.8908) (5.3216, 10.9172) (5.3234, 10.9437) (5.3252, 10.9702) (5.3267, 10.9968) (5.3281, 11.0234) (5.3294, 11.0501) (5.3305, 11.0768) (5.3315, 11.1036) (5.3323, 11.1304) (5.333, 11.1573) (5.3335, 11.1842) (5.3339, 11.2111) (5.3342, 11.2381) (5.3343, 11.2651) (5.3343, 11.2922) (5.3342, 11.3193) (5.3339, 11.3465) (5.3335, 11.3736) (5.3329, 11.4009) (5.3322, 11.4281) (5.3314, 11.4554) (5.3304, 11.4828) (5.3293, 11.5102) (5.3281, 11.5376) (5.3268, 11.565) (5.3253, 11.5925) (5.3237, 11.62) (5.322, 11.6475) (5.3201, 11.6751) (5.3181, 11.7027) (5.316, 11.7304) (5.3138, 11.758) (5.3114, 11.7857) (5.3089, 11.8134) (5.3068, 11.8356) (5.3052, 11.8523) (5.3041, 11.8634) (5.3035, 11.869) knots 0 0 0 0 0 0 0.01428571 0.02857143 0.04285714 0.05714286 0.07142857 0.08571429 0.1 0.11428571 0.12857143 0.14285714 0.15714286 0.17142857 0.18571429 0.2 0.21428571 0.22857143 0.24285714 0.25714286 0.27142857 0.28571429 0.3 0.31428571 0.32857143 0.34285714 0.35714286 0.37142857 0.38571429 0.4 0.41428571 0.42857143 0.44285714 0.45714286 0.47142857 0.48571429 0.5 0.51428571 0.52857143 0.54285714 0.55714286 0.57142857 0.58571429 0.6 0.61428571 0.62857143 0.64285714 0.65714286 0.67142857 0.68571429 0.7 0.71428571 0.72857143 0.74285714 0.75714286 0.77142857 0.78571429 0.8 0.81428571 0.82857143 0.84285714 0.85714286 0.87142857 0.88571429 0.9 0.91428571 0.92857143 0.94285714 0.95714286 0.97142857 0.98571429 1 1 1 1 1 1
  arc A23 (5.3035, 11.869) -> (4.6425, 12.1428) centre (0, 0) ccw
  spline S11 degree 5 poles (4.6425, 12.1428) (4.6382, 12.1392) (4.6295, 12.1322) (4.6166, 12.1215) (4.5994, 12.1073) (4.578, 12.0895) (4.5568, 12.0716) (4.5356, 12.0536) (4.5146, 12.0356) (4.4937, 12.0174) (4.4729, 11.9993) (4.4522, 11.981) (4.4316, 11.9627) (4.4111, 11.9443) (4.3907, 11.9259) (4.3705, 11.9073) (4.3504, 11.8887) (4.3304, 11.8701) (4.3105, 11.8514) (4.2907, 11.8326) (4.2711, 11.8137) (4.2515, 11.7948) (4.2321, 11.7758) (4.2129, 11.7567) (4.1937, 11.7376) (4.1747, 11.7184) (4.1558, 11.6991) (4.137, 11.6798) (4.1184, 11.6604) (4.0999, 11.6409) (4.0815, 11.6213) (4.0633, 11.6017) (4.0452, 11.582) (4.0272, 11.5623) (4.0094, 11.5425) (3.9917, 11.5226) (3.9741, 11.5026) (3.9567, 11.4826) (3.9395, 11.4625) (3.9223, 11.4423) (3.9054, 11.4221) (3.8886, 11.4017) (3.8719, 11.3814) (3.8554, 11.3609) (3.8391, 11.3404) (3.8229, 11.3197) (3.8068, 11.2991) (3.791, 11.2783) (3.7753, 11.2575) (3.7597, 11.2366) (3.7444, 11.2156) (3.7292, 11.1946) (3.7143, 11.1734) (3.6995, 11.1522) (3.6849, 11.1309) (3.6705, 11.1095) (3.6563, 11.088) (3.6422, 11.0665) (3.6284, 11.0449) (3.6147, 11.0232) (3.6013, 11.0014) (3.5883, 10.9795) (3.5755, 10.9575) (3.563, 10.9353) (3.5508, 10.913) (3.5389, 10.8907) (3.527, 10.8683) (3.5154, 10.8459) (3.5039, 10.8233) (3.4929, 10.8007) (3.4826, 10.7777) (3.475, 10.7591) (3.4699, 10.745) (3.4667, 10.7355) (3.4651, 10.7307) knots -1 -1 -1 -1 -1 -1 -0.98571429 -0.97142857 -0.95714286 -0.94285714 -0.92857143 -0.91428571 -0.9 -0.88571429 -0.87142857 -0.85714286 -0.84285714 -0.82857143 -0.81428571 -0.8 -0.78571429 -0.77142857 -0.75714286 -0.74285714 -0.72857143 -0.71428571 -0.7 -0.68571429 -0.67142857 -0.65714286 -0.64285714 -0.62857143 -0.61428571 -0.6 -0.58571429 -0.57142857 -0.55714286 -0.54285714 -0.52857143 -0.51428571 -0.5 -0.48571429 -0.47142857 -0.45714286 -0.44285714 -0.42857143 -0.41428571 -0.4 -0.38571429 -0.37142857 -0.35714286 -0.34285714 -0.32857143 -0.31428571 -0.3 -0.28571429 -0.27142857 -0.25714286 -0.24285714 -0.22857143 -0.21428571 -0.2 -0.18571429 -0.17142857 -0.15714286 -0.14285714 -0.12857143 -0.11428571 -0.1 -0.08571429 -0.07142857 -0.05714286 -0.04285714 -0.02857143 -0.01428571 0 0 0 0 0 0
  line L11 (3.4651, 10.7307) -> (3.4531, 10.6936)
  arc A24 (2.8452, 10.3658) -> (3.4531, 10.6936) centre (2.9775, 10.848) ccw
  arc A25 (2.8452, 10.3658) -> (2.7189, 10.3996) centre (0, 0) ccw
  arc A26 (2.3564, 10.9875) -> (2.7189, 10.3996) centre (2.8454, 10.8834) ccw
  line L12 (2.3564, 10.9875) -> (2.3645, 11.0256)
  spline S12 degree 5 poles (2.3645, 11.0256) (2.3655, 11.0305) (2.3675, 11.0404) (2.3701, 11.0552) (2.3729, 11.0751) (2.3754, 11.1001) (2.3772, 11.1253) (2.3785, 11.1505) (2.3797, 11.1757) (2.3806, 11.201) (2.3814, 11.2264) (2.382, 11.2518) (2.3823, 11.2772) (2.3822, 11.3027) (2.3818, 11.3282) (2.3811, 11.3537) (2.3802, 11.3793) (2.379, 11.405) (2.3776, 11.4307) (2.376, 11.4564) (2.3742, 11.4821) (2.3722, 11.5078) (2.3701, 11.5336) (2.3677, 11.5594) (2.3651, 11.5852) (2.3623, 11.611) (2.3593, 11.6369) (2.3561, 11.6628) (2.3527, 11.6887) (2.3492, 11.7146) (2.3455, 11.7406) (2.3416, 11.7665) (2.3375, 11.7925) (2.3333, 11.8185) (2.3289, 11.8445) (2.3243, 11.8705) (2.3196, 11.8965) (2.3147, 11.9226) (2.3096, 11.9486) (2.3044, 11.9747) (2.299, 12.0007) (2.2935, 12.0268) (2.2878, 12.0529) (2.282, 12.079) (2.276, 12.1051) (2.2698, 12.1312) (2.2636, 12.1574) (2.2571, 12.1835) (2.2505, 12.2096) (2.2438, 12.2358) (2.2369, 12.2619) (2.2299, 12.288) (2.2227, 12.3142) (2.2154, 12.3403) (2.208, 12.3665) (2.2004, 12.3927) (2.1927, 12.4188) (2.1848, 12.445) (2.1768, 12.4711) (2.1687, 12.4973) (2.1604, 12.5235) (2.152, 12.5496) (2.1435, 12.5758) (2.1348, 12.6019) (2.126, 12.6281) (2.1171, 12.6542) (2.108, 12.6804) (2.0988, 12.7065) (2.0895, 12.7327) (2.08, 12.7588) (2.0705, 12.785) (2.0627, 12.8059) (2.0568, 12.8215) (2.0528, 12.832) (2.0509, 12.8372) knots 0 0 0 0 0 0 0.01428571 0.02857143 0.04285714 0.05714286 0.07142857 0.08571429 0.1 0.11428571 0.12857143 0.14285714 0.15714286 0.17142857 0.18571429 0.2 0.21428571 0.22857143 0.24285714 0.25714286 0.27142857 0.28571429 0.3 0.31428571 0.32857143 0.34285714 0.35714286 0.37142857 0.38571429 0.4 0.41428571 0.42857143 0.44285714 0.45714286 0.47142857 0.48571429 0.5 0.51428571 0.52857143 0.54285714 0.55714286 0.57142857 0.58571429 0.6 0.61428571 0.62857143 0.64285714 0.65714286 0.67142857 0.68571429 0.7 0.71428571 0.72857143 0.74285714 0.75714286 0.77142857 0.78571429 0.8 0.81428571 0.82857143 0.84285714 0.85714286 0.87142857 0.88571429 0.9 0.91428571 0.92857143 0.94285714 0.95714286 0.97142857 0.98571429 1 1 1 1 1 1
  arc A27 (2.0509, 12.8372) -> (1.3415, 12.9306) centre (0, 0) ccw
  spline S13 degree 5 poles (1.3415, 12.9306) (1.3383, 12.9261) (1.3317, 12.917) (1.322, 12.9034) (1.3091, 12.8852) (1.2931, 12.8624) (1.2772, 12.8396) (1.2614, 12.8168) (1.2457, 12.7939) (1.2302, 12.771) (1.2148, 12.7481) (1.1995, 12.7251) (1.1844, 12.702) (1.1694, 12.679) (1.1545, 12.6559) (1.1397, 12.6328) (1.1251, 12.6096) (1.1106, 12.5864) (1.0962, 12.5632) (1.082, 12.5399) (1.0679, 12.5166) (1.054, 12.4933) (1.0401, 12.4699) (1.0265, 12.4465) (1.0129, 12.423) (0.9995, 12.3996) (0.9862, 12.3761) (0.9731, 12.3525) (0.9601, 12.329) (0.9473, 12.3054) (0.9346, 12.2817) (0.9221, 12.2581) (0.9097, 12.2344) (0.8974, 12.2106) (0.8853, 12.1869) (0.8734, 12.1631) (0.8616, 12.1392) (0.85, 12.1154) (0.8385, 12.0915) (0.8272, 12.0676) (0.8161, 12.0436) (0.8051, 12.0197) (0.7943, 11.9957) (0.7836, 11.9716) (0.7731, 11.9476) (0.7628, 11.9235) (0.7527, 11.8993) (0.7428, 11.8752) (0.733, 11.851) (0.7234, 11.8268) (0.714, 11.8026) (0.7048, 11.7783) (0.6958, 11.754) (0.687, 11.7297) (0.6785, 11.7053) (0.6701, 11.6809) (0.6619, 11.6565) (0.6539, 11.6321) (0.6461, 11.6076) (0.6386, 11.5832) (0.6313, 11.5586) (0.6243, 11.5341) (0.6177, 11.5095) (0.6114, 11.4849) (0.6053, 11.4602) (0.5996, 11.4355) (0.5939, 11.4108) (0.5885, 11.3861) (0.5833, 11.3614) (0.5785, 11.3367) (0.5744, 11.3119) (0.572, 11.2919) (0.5706, 11.2769) (0.57, 11.2669) (0.5697, 11.2619) knots -1 -1 -1 -1 -1 -1 -0.98571429 -0.97142857 -0.95714286 -0.94285714 -0.92857143 -0.91428571 -0.9 -0.88571429 -0.87142857 -0.85714286 -0.84285714 -0.82857143 -0.81428571 -0.8 -0.78571429 -0.77142857 -0.75714286 -0.74285714 -0.72857143 -0.71428571 -0.7 -0.68571429 -0.67142857 -0.65714286 -0.64285714 -0.62857143 -0.61428571 -0.6 -0.58571429 -0.57142857 -0.55714286 -0.54285714 -0.52857143 -0.51428571 -0.5 -0.48571429 -0.47142857 -0.45714286 -0.44285714 -0.42857143 -0.41428571 -0.4 -0.38571429 -0.37142857 -0.35714286 -0.34285714 -0.32857143 -0.31428571 -0.3 -0.28571429 -0.27142857 -0.25714286 -0.24285714 -0.22857143 -0.21428571 -0.2 -0.18571429 -0.17142857 -0.15714286 -0.14285714 -0.12857143 -0.11428571 -0.1 -0.08571429 -0.07142857 -0.05714286 -0.04285714 -0.02857143 -0.01428571 0 0 0 0 0 0
  line L13 (0.5697, 11.2619) -> (0.5677, 11.223)
  arc A28 (0.0653, 10.749) -> (0.5677, 11.223) centre (0.0684, 11.249) ccw
  arc A29 (0.0653, 10.749) -> (-0.0653, 10.749) centre (0, 0) ccw
  arc A30 (-0.5677, 11.223) -> (-0.0653, 10.749) centre (-0.0684, 11.249) ccw
  line L14 (-0.5677, 11.223) -> (-0.5697, 11.2619)
  spline S14 degree 5 poles (-0.5697, 11.2619) (-0.57, 11.2669) (-0.5706, 11.2769) (-0.572, 11.2919) (-0.5744, 11.3119) (-0.5785, 11.3367) (-0.5833, 11.3614) (-0.5885, 11.3861) (-0.5939, 11.4108) (-0.5996, 11.4355) (-0.6053, 11.4602) (-0.6114, 11.4849) (-0.6177, 11.5095) (-0.6243, 11.5341) (-0.6313, 11.5586) (-0.6386, 11.5832) (-0.6461, 11.6076) (-0.6539, 11.6321) (-0.6619, 11.6565) (-0.6701, 11.6809) (-0.6785, 11.7053) (-0.687, 11.7297) (-0.6958, 11.754) (-0.7048, 11.7783) (-0.714, 11.8026) (-0.7234, 11.8268) (-0.733, 11.851) (-0.7428, 11.8752) (-0.7527, 11.8993) (-0.7628, 11.9235) (-0.7731, 11.9476) (-0.7836, 11.9716) (-0.7943, 11.9957) (-0.8051, 12.0197) (-0.8161, 12.0436) (-0.8272, 12.0676) (-0.8385, 12.0915) (-0.85, 12.1154) (-0.8616, 12.1392) (-0.8734, 12.1631) (-0.8853, 12.1869) (-0.8974, 12.2106) (-0.9097, 12.2344) (-0.9221, 12.2581) (-0.9346, 12.2817) (-0.9473, 12.3054) (-0.9601, 12.329) (-0.9731, 12.3525) (-0.9862, 12.3761) (-0.9995, 12.3996) (-1.0129, 12.423) (-1.0265, 12.4465) (-1.0401, 12.4699) (-1.054, 12.4933) (-1.0679, 12.5166) (-1.082, 12.5399) (-1.0962, 12.5632) (-1.1106, 12.5864) (-1.1251, 12.6096) (-1.1397, 12.6328) (-1.1545, 12.6559) (-1.1694, 12.679) (-1.1844, 12.702) (-1.1995, 12.7251) (-1.2148, 12.7481) (-1.2302, 12.771) (-1.2457, 12.7939) (-1.2614, 12.8168) (-1.2772, 12.8396) (-1.2931, 12.8624) (-1.3091, 12.8852) (-1.322, 12.9034) (-1.3317, 12.917) (-1.3383, 12.9261) (-1.3415, 12.9306) knots 0 0 0 0 0 0 0.01428571 0.02857143 0.04285714 0.05714286 0.07142857 0.08571429 0.1 0.11428571 0.12857143 0.14285714 0.15714286 0.17142857 0.18571429 0.2 0.21428571 0.22857143 0.24285714 0.25714286 0.27142857 0.28571429 0.3 0.31428571 0.32857143 0.34285714 0.35714286 0.37142857 0.38571429 0.4 0.41428571 0.42857143 0.44285714 0.45714286 0.47142857 0.48571429 0.5 0.51428571 0.52857143 0.54285714 0.55714286 0.57142857 0.58571429 0.6 0.61428571 0.62857143 0.64285714 0.65714286 0.67142857 0.68571429 0.7 0.71428571 0.72857143 0.74285714 0.75714286 0.77142857 0.78571429 0.8 0.81428571 0.82857143 0.84285714 0.85714286 0.87142857 0.88571429 0.9 0.91428571 0.92857143 0.94285714 0.95714286 0.97142857 0.98571429 1 1 1 1 1 1
  arc A31 (-1.3415, 12.9306) -> (-2.0509, 12.8372) centre (0, 0) ccw
  spline S15 degree 5 poles (-2.0509, 12.8372) (-2.0528, 12.832) (-2.0568, 12.8215) (-2.0627, 12.8059) (-2.0705, 12.785) (-2.08, 12.7588) (-2.0895, 12.7327) (-2.0988, 12.7065) (-2.108, 12.6804) (-2.1171, 12.6542) (-2.126, 12.6281) (-2.1348, 12.6019) (-2.1435, 12.5758) (-2.152, 12.5496) (-2.1604, 12.5235) (-2.1687, 12.4973) (-2.1768, 12.4711) (-2.1848, 12.445) (-2.1927, 12.4188) (-2.2004, 12.3927) (-2.208, 12.3665) (-2.2154, 12.3403) (-2.2227, 12.3142) (-2.2299, 12.288) (-2.2369, 12.2619) (-2.2438, 12.2358) (-2.2505, 12.2096) (-2.2571, 12.1835) (-2.2636, 12.1574) (-2.2698, 12.1312) (-2.276, 12.1051) (-2.282, 12.079) (-2.2878, 12.0529) (-2.2935, 12.0268) (-2.299, 12.0007) (-2.3044, 11.9747) (-2.3096, 11.9486) (-2.3147, 11.9226) (-2.3196, 11.8965) (-2.3243, 11.8705) (-2.3289, 11.8445) (-2.3333, 11.8185) (-2.3375, 11.7925) (-2.3416, 11.7665) (-2.3455, 11.7406) (-2.3492, 11.7146) (-2.3527, 11.6887) (-2.3561, 11.6628) (-2.3593, 11.6369) (-2.3623, 11.611) (-2.3651, 11.5852) (-2.3677, 11.5594) (-2.3701, 11.5336) (-2.3722, 11.5078) (-2.3742, 11.4821) (-2.376, 11.4564) (-2.3776, 11.4307) (-2.379, 11.405) (-2.3802, 11.3793) (-2.3811, 11.3537) (-2.3818, 11.3282) (-2.3822, 11.3027) (-2.3823, 11.2772) (-2.382, 11.2518) (-2.3814, 11.2264) (-2.3806, 11.201) (-2.3797, 11.1757) (-2.3785, 11.1505) (-2.3772, 11.1253) (-2.3754, 11.1001) (-2.3729, 11.0751) (-2.3701, 11.0552) (-2.3675, 11.0404) (-2.3655, 11.0305) (-2.3645, 11.0256) knots -1 -1 -1 -1 -1 -1 -0.98571429 -0.97142857 -0.95714286 -0.94285714 -0.92857143 -0.91428571 -0.9 -0.88571429 -0.87142857 -0.85714286 -0.84285714 -0.82857143 -0.81428571 -0.8 -0.78571429 -0.77142857 -0.75714286 -0.74285714 -0.72857143 -0.71428571 -0.7 -0.68571429 -0.67142857 -0.65714286 -0.64285714 -0.62857143 -0.61428571 -0.6 -0.58571429 -0.57142857 -0.55714286 -0.54285714 -0.52857143 -0.51428571 -0.5 -0.48571429 -0.47142857 -0.45714286 -0.44285714 -0.42857143 -0.41428571 -0.4 -0.38571429 -0.37142857 -0.35714286 -0.34285714 -0.32857143 -0.31428571 -0.3 -0.28571429 -0.27142857 -0.25714286 -0.24285714 -0.22857143 -0.21428571 -0.2 -0.18571429 -0.17142857 -0.15714286 -0.14285714 -0.12857143 -0.11428571 -0.1 -0.08571429 -0.07142857 -0.05714286 -0.04285714 -0.02857143 -0.01428571 0 0 0 0 0 0
  line L15 (-2.3645, 11.0256) -> (-2.3564, 10.9875)
  arc A32 (-2.7189, 10.3996) -> (-2.3564, 10.9875) centre (-2.8454, 10.8834) ccw
  arc A33 (-2.7189, 10.3996) -> (-2.8452, 10.3658) centre (0, 0) ccw
  arc A34 (-3.4531, 10.6936) -> (-2.8452, 10.3658) centre (-2.9775, 10.848) ccw
  line L16 (-3.4531, 10.6936) -> (-3.4651, 10.7307)
  spline S16 degree 5 poles (-3.4651, 10.7307) (-3.4667, 10.7355) (-3.4699, 10.745) (-3.475, 10.7591) (-3.4826, 10.7777) (-3.4929, 10.8007) (-3.5039, 10.8233) (-3.5154, 10.8459) (-3.527, 10.8683) (-3.5389, 10.8907) (-3.5508, 10.913) (-3.563, 10.9353) (-3.5755, 10.9575) (-3.5883, 10.9795) (-3.6013, 11.0014) (-3.6147, 11.0232) (-3.6284, 11.0449) (-3.6422, 11.0665) (-3.6563, 11.088) (-3.6705, 11.1095) (-3.6849, 11.1309) (-3.6995, 11.1522) (-3.7143, 11.1734) (-3.7292, 11.1946) (-3.7444, 11.2156) (-3.7597, 11.2366) (-3.7753, 11.2575) (-3.791, 11.2783) (-3.8068, 11.2991) (-3.8229, 11.3197) (-3.8391, 11.3404) (-3.8554, 11.3609) (-3.8719, 11.3814) (-3.8886, 11.4017) (-3.9054, 11.4221) (-3.9223, 11.4423) (-3.9395, 11.4625) (-3.9567, 11.4826) (-3.9741, 11.5026) (-3.9917, 11.5226) (-4.0094, 11.5425) (-4.0272, 11.5623) (-4.0452, 11.582) (-4.0633, 11.6017) (-4.0815, 11.6213) (-4.0999, 11.6409) (-4.1184, 11.6604) (-4.137, 11.6798) (-4.1558, 11.6991) (-4.1747, 11.7184) (-4.1937, 11.7376) (-4.2129, 11.7567) (-4.2321, 11.7758) (-4.2515, 11.7948) (-4.2711, 11.8137) (-4.2907, 11.8326) (-4.3105, 11.8514) (-4.3304, 11.8701) (-4.3504, 11.8887) (-4.3705, 11.9073) (-4.3907, 11.9259) (-4.4111, 11.9443) (-4.4316, 11.9627) (-4.4522, 11.981) (-4.4729, 11.9993) (-4.4937, 12.0174) (-4.5146, 12.0356) (-4.5356, 12.0536) (-4.5568, 12.0716) (-4.578, 12.0895) (-4.5994, 12.1073) (-4.6166, 12.1215) (-4.6295, 12.1322) (-4.6382, 12.1392) (-4.6425, 12.1428) knots 0 0 0 0 0 0 0.01428571 0.02857143 0.04285714 0.05714286 0.07142857 0.08571429 0.1 0.11428571 0.12857143 0.14285714 0.15714286 0.17142857 0.18571429 0.2 0.21428571 0.22857143 0.24285714 0.25714286 0.27142857 0.28571429 0.3 0.31428571 0.32857143 0.34285714 0.35714286 0.37142857 0.38571429 0.4 0.41428571 0.42857143 0.44285714 0.45714286 0.47142857 0.48571429 0.5 0.51428571 0.52857143 0.54285714 0.55714286 0.57142857 0.58571429 0.6 0.61428571 0.62857143 0.64285714 0.65714286 0.67142857 0.68571429 0.7 0.71428571 0.72857143 0.74285714 0.75714286 0.77142857 0.78571429 0.8 0.81428571 0.82857143 0.84285714 0.85714286 0.87142857 0.88571429 0.9 0.91428571 0.92857143 0.94285714 0.95714286 0.97142857 0.98571429 1 1 1 1 1 1
  arc A35 (-4.6425, 12.1428) -> (-5.3035, 11.869) centre (0, 0) ccw
  spline S17 degree 5 poles (-5.3035, 11.869) (-5.3041, 11.8634) (-5.3052, 11.8523) (-5.3068, 11.8356) (-5.3089, 11.8134) (-5.3114, 11.7857) (-5.3138, 11.758) (-5.316, 11.7304) (-5.3181, 11.7027) (-5.3201, 11.6751) (-5.322, 11.6475) (-5.3237, 11.62) (-5.3253, 11.5925) (-5.3268, 11.565) (-5.3281, 11.5376) (-5.3293, 11.5102) (-5.3304, 11.4828) (-5.3314, 11.4554) (-5.3322, 11.4281) (-5.3329, 11.4009) (-5.3335, 11.3736) (-5.3339, 11.3465) (-5.3342, 11.3193) (-5.3343, 11.2922) (-5.3343, 11.2651) (-5.3342, 11.2381) (-5.3339, 11.2111) (-5.3335, 11.1842) (-5.333, 11.1573) (-5.3323, 11.1304) (-5.3315, 11.1036) (-5.3305, 11.0768) (-5.3294, 11.0501) (-5.3281, 11.0234) (-5.3267, 10.9968) (-5.3252, 10.9702) (-5.3234, 10.9437) (-5.3216, 10.9172) (-5.3196, 10.8908) (-5.3174, 10.8644) (-5.3151, 10.8381) (-5.3126, 10.8119) (-5.31, 10.7857) (-5.3072, 10.7595) (-5.3042, 10.7335) (-5.3011, 10.7075) (-5.2978, 10.6815) (-5.2943, 10.6556) (-5.2907, 10.6298) (-5.2869, 10.604) (-5.283, 10.5783) (-5.2788, 10.5527) (-5.2744, 10.5272) (-5.2698, 10.5017) (-5.2651, 10.4763) (-5.2601, 10.451) (-5.255, 10.4258) (-5.2497, 10.4007) (-5.2443, 10.3756) (-5.2386, 10.3506) (-5.2326, 10.3257) (-5.2264, 10.301) (-5.2198, 10.2763) (-5.213, 10.2519) (-5.2059, 10.2275) (-5.1985, 10.2032) (-5.1911, 10.179) (-5.1834, 10.1549) (-5.1756, 10.1309) (-5.1673, 10.1071) (-5.1585, 10.0836) (-5.1506, 10.0651) (-5.1443, 10.0514) (-5.1398, 10.0424) (-5.1376, 10.038) knots -1 -1 -1 -1 -1 -1 -0.98571429 -0.97142857 -0.95714286 -0.94285714 -0.92857143 -0.91428571 -0.9 -0.88571429 -0.87142857 -0.85714286 -0.84285714 -0.82857143 -0.81428571 -0.8 -0.78571429 -0.77142857 -0.75714286 -0.74285714 -0.72857143 -0.71428571 -0.7 -0.68571429 -0.67142857 -0.65714286 -0.64285714 -0.62857143 -0.61428571 -0.6 -0.58571429 -0.57142857 -0.55714286 -0.54285714 -0.52857143 -0.51428571 -0.5 -0.48571429 -0.47142857 -0.45714286 -0.44285714 -0.42857143 -0.41428571 -0.4 -0.38571429 -0.37142857 -0.35714286 -0.34285714 -0.32857143 -0.31428571 -0.3 -0.28571429 -0.27142857 -0.25714286 -0.24285714 -0.22857143 -0.21428571 -0.2 -0.18571429 -0.17142857 -0.15714286 -0.14285714 -0.12857143 -0.11428571 -0.1 -0.08571429 -0.07142857 -0.05714286 -0.04285714 -0.02857143 -0.01428571 0 0 0 0 0 0
  line L17 (-5.1376, 10.038) -> (-5.1199, 10.0032)
  arc A36 (-5.3179, 9.3416) -> (-5.1199, 10.0032) centre (-5.5653, 9.7761) ccw
  arc A37 (-5.3179, 9.3416) -> (-5.4311, 9.2762) centre (0, 0) ccw
  arc A38 (-6.1031, 9.4355) -> (-5.4311, 9.2762) centre (-5.6837, 9.7077) ccw
  line L18 (-6.1031, 9.4355) -> (-6.1244, 9.4682)